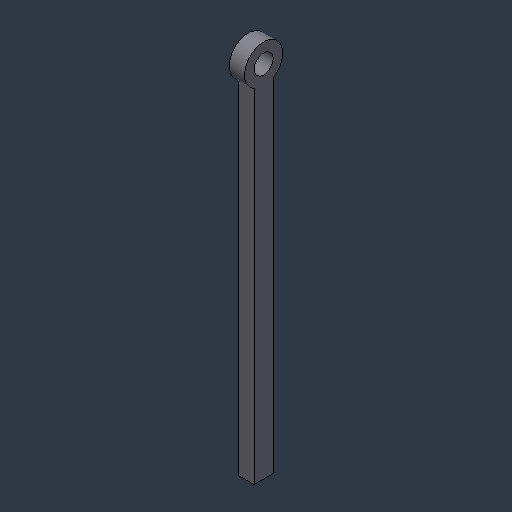
# Autodesk Inventor part: TUBE,CF,ARM
Saved by Autodesk Inventor 2024.3 (Build 283343000, 343)
## iProperties
Category: _
Manager: _
ILogicPurgeVersion: 0.0.0.0
OnSaveVersion: 3.5.0.0
OnSaveAssembly: COREAutomationManager
Created: 2025-03-06
Part Number: TUBE,CF,ARM
Checked By: 00
Engr Approved By: _
User Status: Work In Process
Material: Steel, MS
Description: STANDARD (mm)
Document SubType Name: Modeling
Mfg Approved By: John.Thibert
Designer: John.Thibert
Manufacturer: Standard
Standards Organization: Custom
Mass: 4065.24 g
Surface Area: 772.131 cm^2
Volume: 517.206 cm^3
Density: 7.86 g/cm^3
Appearance: Metal-Steel
CN_MASS: 4.07
CN_SERVICEABLE: _
FIRST_DESCRIPTION: _
SECOND_DESCRIPTION: _
THIRD_DESCRIPTION: _
ModelCat: Uncategorized
MaterialName: Steel, MS
Subject: _
Author: John.Thibert
Keywords: -
Revision Number: A
Autodesk Inventor part; units mm, degrees
ref_plane "YZ Plane" through (0, 0, 0) normal (1, 0, 0) x (0, 1, 0)
ref_plane "XZ Plane" through (0, 0, 0) normal (0, 1, 0) x (-1, 0, 0)
ref_plane "XY Plane" through (0, 0, 0) normal (0, 0, 1) x (1, 0, 0)
sketch "Sketch2" plane through (0, 0, 0) normal (1, 0, 0) x (0, 1, 0)
  circle A0 centre (0, 0) radius 15.875
  arc A1 (-27.4963, -15.875) -> (-27.4963, 15.875) centre (0, 0) ccw
  line L0 (-27.4963, 15.875) -> (-596.9, 15.875)
  line L1 (-596.9, 15.875) -> (-596.9, -15.875)
  line L2 (-596.9, -15.875) -> (-27.4963, -15.875)
  dimension "d0" = 31.75
  dimension "d1" = 31.75
  dimension "d2" = 31.75
  dimension "d3" = 596.9
  constraints: 6 end point, 2 centre point, 2 coincident, 2 point on circle, 1 horizontal, 1 parallel, 1 perpendicular, 1 vertical
  measures "d0" diameter of A0
  measures "d1" distance of L0.end L1.end
  measures "d2" radius of A1
  measures "d3" distance from line of L1 A0.centre
extrude "Extrusion1" add sketch "Sketch2" along normal mid plane 25.4
body "Solid1"
